Autodesk Inventor part; units mm, degrees
(part 6 of 8)
  spline S746 degree 2 poles (-18.7329, -20.1182) (-18.7329, -19.7747) (-18.2437, -19.289) (-17.9037, -19.289) knots 0 0 0 1 2 2 2
  line L2512 (-18.7329, -20.1182) -> (-18.7329, -19.7747) construction
  line L2513 (-18.7329, -19.7747) -> (-18.2437, -19.289) construction
  line L2514 (-18.2437, -19.289) -> (-17.9037, -19.289) construction
  line L2515 (-17.9037, -19.289) -> (-16.8664, -19.289)
  spline S747 degree 2 poles (-16.8664, -19.289) (-16.6582, -19.289) (-16.6582, -19.4972) knots 0 0 0 1 1 1
  line L2516 (-16.8664, -19.289) -> (-16.6582, -19.289) construction
  line L2517 (-16.6582, -19.289) -> (-16.6582, -19.4972) construction
  line L2518 (-16.6582, -19.4972) -> (-16.6582, -21.3602)
  spline S748 degree 2 poles (-16.6582, -21.3602) (-16.6582, -21.6725) (-16.3668, -21.7974) knots 0 0 0 1 1 1
  line L2519 (-16.6582, -21.3602) -> (-16.6582, -21.6725) construction
  line L2520 (-16.6582, -21.6725) -> (-16.3668, -21.7974) construction
  spline S749 degree 2 poles (-16.3668, -21.7974) (-16.2384, -21.8494) (-16.2384, -21.9812) knots 0 0 0 1 1 1
  line L2521 (-16.3668, -21.7974) -> (-16.2384, -21.8494) construction
  line L2522 (-16.2384, -21.8494) -> (-16.2384, -21.9812) construction
  spline S750 degree 2 poles (-16.2384, -21.9812) (-16.2384, -22.068) (-16.3564, -22.1998) (-16.4431, -22.1998) knots 0 0 0 1 2 2 2
  line L2523 (-16.2384, -21.9812) -> (-16.2384, -22.068) construction
  line L2524 (-16.2384, -22.068) -> (-16.3564, -22.1998) construction
  line L2525 (-16.3564, -22.1998) -> (-16.4431, -22.1998) construction
  spline S751 degree 2 poles (-16.4431, -22.1998) (-16.4882, -22.1998) (-16.5333, -22.179) knots 0 0 0 1 1 1
  line L2526 (-16.4431, -22.1998) -> (-16.4882, -22.1998) construction
  line L2527 (-16.4882, -22.1998) -> (-16.5333, -22.179) construction
  spline S752 degree 2 poles (-16.5333, -22.179) (-16.7415, -22.0888) (-16.8699, -21.9222) knots 0 0 0 1 1 1
  line L2528 (-16.5333, -22.179) -> (-16.7415, -22.0888) construction
  line L2529 (-16.7415, -22.0888) -> (-16.8699, -21.9222) construction
  spline S753 degree 2 poles (-16.8699, -21.9222) (-17.1197, -22.1963) (-17.4874, -22.1963) knots 0 0 0 1 1 1
  line L2530 (-16.8699, -21.9222) -> (-17.1197, -22.1963) construction
  line L2531 (-17.1197, -22.1963) -> (-17.4874, -22.1963) construction
  spline S754 degree 2 poles (-13.9591, -22.1963) (-14.1673, -22.1963) (-14.1673, -21.9882) knots 0 0 0 1 1 1
  line L2532 (-13.9591, -22.1963) -> (-14.1673, -22.1963) construction
  line L2533 (-14.1673, -22.1963) -> (-14.1673, -21.9882) construction
  line L2534 (-14.1673, -21.9882) -> (-14.1673, -20.1217)
  spline S755 degree 2 poles (-14.1673, -20.1217) (-14.1673, -19.9517) (-14.4101, -19.7053) (-14.5801, -19.7053) knots 0 0 0 1 2 2 2
  line L2535 (-14.1673, -20.1217) -> (-14.1673, -19.9517) construction
  line L2536 (-14.1673, -19.9517) -> (-14.4101, -19.7053) construction
  line L2537 (-14.4101, -19.7053) -> (-14.5801, -19.7053) construction
  spline S756 degree 2 poles (-15.4093, -21.9882) (-15.4093, -22.1963) (-15.6174, -22.1963) knots 0 0 0 1 1 1
  line L2538 (-15.4093, -21.9882) -> (-15.4093, -22.1963) construction
  line L2539 (-15.4093, -22.1963) -> (-15.6174, -22.1963) construction
  spline S757 degree 2 poles (-15.6174, -22.1963) (-15.8256, -22.1963) (-15.8256, -21.9882) knots 0 0 0 1 1 1
  line L2540 (-15.6174, -22.1963) -> (-15.8256, -22.1963) construction
  line L2541 (-15.8256, -22.1963) -> (-15.8256, -21.9882) construction
  line L2542 (-15.8256, -21.9882) -> (-15.8256, -19.4972)
  spline S758 degree 2 poles (-15.8256, -19.4972) (-15.8256, -19.289) (-15.6174, -19.289) knots 0 0 0 1 1 1
  line L2543 (-15.8256, -19.4972) -> (-15.8256, -19.289) construction
  line L2544 (-15.8256, -19.289) -> (-15.6174, -19.289) construction
  line L2545 (-15.6174, -19.289) -> (-14.5801, -19.289)
  spline S759 degree 2 poles (-14.5801, -19.289) (-14.2366, -19.289) (-13.7509, -19.7747) (-13.7509, -20.1182) knots 0 0 0 1 2 2 2
  line L2546 (-14.5801, -19.289) -> (-14.2366, -19.289) construction
  line L2547 (-14.2366, -19.289) -> (-13.7509, -19.7747) construction
  line L2548 (-13.7509, -19.7747) -> (-13.7509, -20.1182) construction
  line L2549 (-13.7509, -20.1182) -> (-13.7509, -21.9882)
  spline S760 degree 2 poles (-13.7509, -21.9882) (-13.7509, -22.1963) (-13.9591, -22.1963) knots 0 0 0 1 1 1
  line L2550 (-13.7509, -21.9882) -> (-13.7509, -22.1963) construction
  line L2551 (-13.7509, -22.1963) -> (-13.9591, -22.1963) construction
  spline S761 degree 2 poles (-9.1784, -22.1963) (-9.5184, -22.1963) (-10.011, -21.7106) (-10.011, -21.3672) knots 0 0 0 1 2 2 2
  line L2552 (-9.1784, -22.1963) -> (-9.5184, -22.1963) construction
  line L2553 (-9.5184, -22.1963) -> (-10.011, -21.7106) construction
  line L2554 (-10.011, -21.7106) -> (-10.011, -21.3672) construction
  line L2555 (-10.011, -21.3672) -> (-10.011, -20.1182)
  spline S762 degree 2 poles (-10.011, -20.1182) (-10.011, -19.7747) (-9.5184, -19.289) (-9.1784, -19.289) knots 0 0 0 1 2 2 2
  line L2556 (-10.011, -20.1182) -> (-10.011, -19.7747) construction
  line L2557 (-10.011, -19.7747) -> (-9.5184, -19.289) construction
  line L2558 (-9.5184, -19.289) -> (-9.1784, -19.289) construction
  line L2559 (-9.1784, -19.289) -> (-8.5573, -19.289)
  spline S763 degree 2 poles (-8.5573, -19.289) (-8.3492, -19.289) (-8.3492, -19.4972) knots 0 0 0 1 1 1
  line L2560 (-8.5573, -19.289) -> (-8.3492, -19.289) construction
  line L2561 (-8.3492, -19.289) -> (-8.3492, -19.4972) construction
  spline S764 degree 2 poles (-8.3492, -19.4972) (-8.3492, -19.7053) (-8.5573, -19.7053) knots 0 0 0 1 1 1
  line L2562 (-8.3492, -19.4972) -> (-8.3492, -19.7053) construction
  line L2563 (-8.3492, -19.7053) -> (-8.5573, -19.7053) construction
  line L2564 (-8.5573, -19.7053) -> (-9.1784, -19.7053)
  spline S765 degree 2 poles (-9.1784, -19.7053) (-9.3484, -19.7053) (-9.5947, -19.9517) (-9.5947, -20.1217) knots 0 0 0 1 2 2 2
  line L2565 (-9.1784, -19.7053) -> (-9.3484, -19.7053) construction
  line L2566 (-9.3484, -19.7053) -> (-9.5947, -19.9517) construction
  line L2567 (-9.5947, -19.9517) -> (-9.5947, -20.1217) construction
  line L2568 (-9.5947, -20.1217) -> (-9.5947, -21.3637)
  spline S766 degree 2 poles (-9.5947, -21.3637) (-9.5947, -21.5337) (-9.3484, -21.78) (-9.1784, -21.78) knots 0 0 0 1 2 2 2
  line L2569 (-9.5947, -21.3637) -> (-9.5947, -21.5337) construction
  line L2570 (-9.5947, -21.5337) -> (-9.3484, -21.78) construction
  line L2571 (-9.3484, -21.78) -> (-9.1784, -21.78) construction
  line L2572 (-9.1784, -21.78) -> (-8.5573, -21.78)
  spline S767 degree 2 poles (-8.5573, -21.78) (-8.3492, -21.78) (-8.3492, -21.9882) knots 0 0 0 1 1 1
  line L2573 (-8.5573, -21.78) -> (-8.3492, -21.78) construction
  line L2574 (-8.3492, -21.78) -> (-8.3492, -21.9882) construction
  spline S768 degree 2 poles (-8.3492, -21.9882) (-8.3492, -22.1963) (-8.5573, -22.1963) knots 0 0 0 1 1 1
  line L2575 (-8.3492, -21.9882) -> (-8.3492, -22.1963) construction
  line L2576 (-8.3492, -22.1963) -> (-8.5573, -22.1963) construction
  line L2577 (-8.5573, -22.1963) -> (-9.1784, -22.1963)
  spline S769 degree 2 poles (-17.474, -28.914) (-17.2173, -28.914) (-16.853, -28.5497) (-16.853, -28.293) knots 0 0 0 1 2 2 2
  line L2578 (-17.474, -28.914) -> (-17.2173, -28.914) construction
  line L2579 (-17.2173, -28.914) -> (-16.853, -28.5497) construction
  line L2580 (-16.853, -28.5497) -> (-16.853, -28.293) construction
  line L2581 (-16.853, -28.293) -> (-16.853, -26.2149)
  spline S770 degree 2 poles (-16.853, -26.2149) (-16.853, -25.9581) (-17.2173, -25.5939) (-17.474, -25.5939) knots 0 0 0 1 2 2 2
  line L2582 (-16.853, -26.2149) -> (-16.853, -25.9581) construction
  line L2583 (-16.853, -25.9581) -> (-17.2173, -25.5939) construction
  line L2584 (-17.2173, -25.5939) -> (-17.474, -25.5939) construction
  line L2585 (-17.474, -29.3303) -> (-18.7195, -29.3303)
  spline S771 degree 2 poles (-18.7195, -29.3303) (-18.8028, -29.3303) (-18.9277, -29.2054) (-18.9277, -29.1222) knots 0 0 0 1 2 2 2
  line L2586 (-18.7195, -29.3303) -> (-18.8028, -29.3303) construction
  line L2587 (-18.8028, -29.3303) -> (-18.9277, -29.2054) construction
  line L2588 (-18.9277, -29.2054) -> (-18.9277, -29.1222) construction
  line L2589 (-18.9277, -29.1222) -> (-18.9277, -25.3857)
  spline S772 degree 2 poles (-18.9277, -25.3857) (-18.9277, -25.3024) (-18.8028, -25.1775) (-18.7195, -25.1775) knots 0 0 0 1 2 2 2
  line L2590 (-18.9277, -25.3857) -> (-18.9277, -25.3024) construction
  line L2591 (-18.9277, -25.3024) -> (-18.8028, -25.1775) construction
  line L2592 (-18.8028, -25.1775) -> (-18.7195, -25.1775) construction
  line L2593 (-18.7195, -25.1775) -> (-17.474, -25.1775)
  spline S773 degree 2 poles (-17.474, -25.1775) (-17.0438, -25.1775) (-16.4367, -25.7881) (-16.4367, -26.2149) knots 0 0 0 1 2 2 2
  line L2594 (-17.474, -25.1775) -> (-17.0438, -25.1775) construction
  line L2595 (-17.0438, -25.1775) -> (-16.4367, -25.7881) construction
  line L2596 (-16.4367, -25.7881) -> (-16.4367, -26.2149) construction
  line L2597 (-16.4367, -26.2149) -> (-16.4367, -28.293)
  spline S774 degree 2 poles (-16.4367, -28.293) (-16.4367, -28.7232) (-17.0438, -29.3303) (-17.474, -29.3303) knots 0 0 0 1 2 2 2
  line L2598 (-16.4367, -28.293) -> (-16.4367, -28.7232) construction
  line L2599 (-16.4367, -28.7232) -> (-17.0438, -29.3303) construction
  line L2600 (-17.0438, -29.3303) -> (-17.474, -29.3303) construction
  spline S775 degree 2 poles (-19.6338, -32.3113) (-19.4256, -32.3113) (-19.4256, -32.5194) knots 0 0 0 1 1 1
  line L2601 (-19.6338, -32.3113) -> (-19.4256, -32.3113) construction
  line L2602 (-19.4256, -32.3113) -> (-19.4256, -32.5194) construction
  spline S776 degree 2 poles (-19.4256, -32.5194) (-19.4256, -32.7276) (-19.6338, -32.7276) knots 0 0 0 1 1 1
  line L2603 (-19.4256, -32.5194) -> (-19.4256, -32.7276) construction
  line L2604 (-19.4256, -32.7276) -> (-19.6338, -32.7276) construction
  spline S777 degree 2 poles (-21.0874, -34.601) (-21.0874, -34.8092) (-21.2956, -34.8092) knots 0 0 0 1 1 1
  line L2605 (-21.0874, -34.601) -> (-21.0874, -34.8092) construction
  line L2606 (-21.0874, -34.8092) -> (-21.2956, -34.8092) construction
  spline S778 degree 2 poles (-21.2956, -34.8092) (-21.5037, -34.8092) (-21.5037, -34.601) knots 0 0 0 1 1 1
  line L2607 (-21.2956, -34.8092) -> (-21.5037, -34.8092) construction
  line L2608 (-21.5037, -34.8092) -> (-21.5037, -34.601) construction
  line L2609 (-21.5037, -34.601) -> (-21.5037, -30.8646)
  spline S779 degree 2 poles (-21.5037, -30.8646) (-21.5037, -30.6564) (-21.2956, -30.6564) knots 0 0 0 1 1 1
  line L2610 (-21.5037, -30.8646) -> (-21.5037, -30.6564) construction
  line L2611 (-21.5037, -30.6564) -> (-21.2956, -30.6564) construction
  line L2612 (-21.2956, -30.6564) -> (-19.6338, -30.6564)
  spline S780 degree 2 poles (-19.6338, -30.6564) (-19.4256, -30.6564) (-19.4256, -30.8646) knots 0 0 0 1 1 1
  line L2613 (-19.6338, -30.6564) -> (-19.4256, -30.6564) construction
  line L2614 (-19.4256, -30.6564) -> (-19.4256, -30.8646) construction
  spline S781 degree 2 poles (-19.4256, -30.8646) (-19.4256, -31.0727) (-19.6338, -31.0727) knots 0 0 0 1 1 1
  line L2615 (-19.4256, -30.8646) -> (-19.4256, -31.0727) construction
  line L2616 (-19.4256, -31.0727) -> (-19.6338, -31.0727) construction
  line L2617 (9.3223, -22.1486) -> (8.2849, -22.1486)
  spline S782 degree 2 poles (8.2849, -22.1486) (7.9449, -22.1486) (7.4558, -21.6629) (7.4558, -21.3195) knots 0 0 0 1 2 2 2
  line L2618 (8.2849, -22.1486) -> (7.9449, -22.1486) construction
  line L2619 (7.9449, -22.1486) -> (7.4558, -21.6629) construction
  line L2620 (7.4558, -21.6629) -> (7.4558, -21.3195) construction
  line L2621 (7.4558, -21.3195) -> (7.4558, -19.4495)
  spline S783 degree 2 poles (7.4558, -19.4495) (7.4558, -19.2413) (7.6639, -19.2413) knots 0 0 0 1 1 1
  line L2622 (7.4558, -19.4495) -> (7.4558, -19.2413) construction
  line L2623 (7.4558, -19.2413) -> (7.6639, -19.2413) construction
  spline S784 degree 2 poles (7.6639, -19.2413) (7.8721, -19.2413) (7.8721, -19.4495) knots 0 0 0 1 1 1
  line L2624 (7.6639, -19.2413) -> (7.8721, -19.2413) construction
  line L2625 (7.8721, -19.2413) -> (7.8721, -19.4495) construction
  line L2626 (7.8721, -19.4495) -> (7.8721, -21.316)
  spline S785 degree 2 poles (7.8721, -21.316) (7.8721, -21.486) (8.1149, -21.7323) (8.2849, -21.7323) knots 0 0 0 1 2 2 2
  line L2627 (7.8721, -21.316) -> (7.8721, -21.486) construction
  line L2628 (7.8721, -21.486) -> (8.1149, -21.7323) construction
  line L2629 (8.1149, -21.7323) -> (8.2849, -21.7323) construction
  spline S786 degree 2 poles (9.1141, -19.4495) (9.1141, -19.2413) (9.3223, -19.2413) knots 0 0 0 1 1 1
  line L2630 (9.1141, -19.4495) -> (9.1141, -19.2413) construction
  line L2631 (9.1141, -19.2413) -> (9.3223, -19.2413) construction
  spline S787 degree 2 poles (9.3223, -19.2413) (9.5304, -19.2413) (9.5304, -19.4495) knots 0 0 0 1 1 1
  line L2632 (9.3223, -19.2413) -> (9.5304, -19.2413) construction
  line L2633 (9.5304, -19.2413) -> (9.5304, -19.4495) construction
  line L2634 (9.5304, -19.4495) -> (9.5304, -21.9405)
  spline S788 degree 2 poles (9.5304, -21.9405) (9.5304, -22.1486) (9.3223, -22.1486) knots 0 0 0 1 1 1
  line L2635 (9.5304, -21.9405) -> (9.5304, -22.1486) construction
  line L2636 (9.5304, -22.1486) -> (9.3223, -22.1486) construction
  spline S789 degree 2 poles (15.345, -22.1486) (15.1369, -22.1486) (15.1369, -21.9405) knots 0 0 0 1 1 1
  line L2637 (15.345, -22.1486) -> (15.1369, -22.1486) construction
  line L2638 (15.1369, -22.1486) -> (15.1369, -21.9405) construction
  spline S790 degree 2 poles (14.4777, -21.0211) (14.3979, -21.1356) (14.3077, -21.1356) knots 0 0 0 1 1 1
  line L2639 (14.4777, -21.0211) -> (14.3979, -21.1356) construction
  line L2640 (14.3979, -21.1356) -> (14.3077, -21.1356) construction
  spline S791 degree 2 poles (14.3077, -21.1356) (14.2175, -21.1356) (14.1377, -21.0211) knots 0 0 0 1 1 1
  line L2641 (14.3077, -21.1356) -> (14.2175, -21.1356) construction
  line L2642 (14.2175, -21.1356) -> (14.1377, -21.0211) construction
  spline S792 degree 2 poles (13.4785, -21.9405) (13.4785, -22.1486) (13.2704, -22.1486) knots 0 0 0 1 1 1
  line L2643 (13.4785, -21.9405) -> (13.4785, -22.1486) construction
  line L2644 (13.4785, -22.1486) -> (13.2704, -22.1486) construction
  spline S793 degree 2 poles (13.2704, -22.1486) (13.0622, -22.1486) (13.0622, -21.9405) knots 0 0 0 1 1 1
  line L2645 (13.2704, -22.1486) -> (13.0622, -22.1486) construction
  line L2646 (13.0622, -22.1486) -> (13.0622, -21.9405) construction
  line L2647 (13.0622, -21.9405) -> (13.0622, -19.446)
  spline S794 degree 2 poles (13.0622, -19.446) (13.0622, -19.2066) (13.2461, -19.2066) knots 0 0 0 1 1 1
  line L2648 (13.0622, -19.446) -> (13.0622, -19.2066) construction
  line L2649 (13.0622, -19.2066) -> (13.2461, -19.2066) construction
  spline S795 degree 2 poles (13.2461, -19.2066) (13.3536, -19.2066) (13.4404, -19.3281) knots 0 0 0 1 1 1
  line L2650 (13.2461, -19.2066) -> (13.3536, -19.2066) construction
  line L2651 (13.3536, -19.2066) -> (13.4404, -19.3281) construction
  spline S796 degree 2 poles (15.175, -19.3281) (15.2618, -19.2066) (15.3693, -19.2066) knots 0 0 0 1 1 1
  line L2652 (15.175, -19.3281) -> (15.2618, -19.2066) construction
  line L2653 (15.2618, -19.2066) -> (15.3693, -19.2066) construction
  spline S797 degree 2 poles (15.3693, -19.2066) (15.5532, -19.2066) (15.5532, -19.446) knots 0 0 0 1 1 1
  line L2654 (15.3693, -19.2066) -> (15.5532, -19.2066) construction
  line L2655 (15.5532, -19.2066) -> (15.5532, -19.446) construction
  line L2656 (15.5532, -19.446) -> (15.5532, -21.9405)
  spline S798 degree 2 poles (15.5532, -21.9405) (15.5532, -22.1486) (15.345, -22.1486) knots 0 0 0 1 1 1
  line L2657 (15.5532, -21.9405) -> (15.5532, -22.1486) construction
  line L2658 (15.5532, -22.1486) -> (15.345, -22.1486) construction
  spline S799 degree 2 poles (6.716, -26.7765) (6.886, -26.7765) (7.1288, -26.5301) (7.1288, -26.3601) knots 0 0 0 1 2 2 2
  line L2659 (6.716, -26.7765) -> (6.886, -26.7765) construction
  line L2660 (6.886, -26.7765) -> (7.1288, -26.5301) construction
  line L2661 (7.1288, -26.5301) -> (7.1288, -26.3601) construction
  line L2662 (7.1288, -26.3601) -> (7.1288, -25.1181)
  spline S800 degree 2 poles (7.1288, -25.1181) (7.1288, -24.9481) (6.886, -24.7018) (6.716, -24.7018) knots 0 0 0 1 2 2 2
  line L2663 (7.1288, -25.1181) -> (7.1288, -24.9481) construction
  line L2664 (7.1288, -24.9481) -> (6.886, -24.7018) construction
  line L2665 (6.886, -24.7018) -> (6.716, -24.7018) construction
  line L2666 (6.716, -24.7018) -> (6.2997, -24.7018)
  spline S801 degree 2 poles (6.2997, -24.7018) (6.1297, -24.7018) (5.8868, -24.9481) (5.8868, -25.1181) knots 0 0 0 1 2 2 2
  line L2667 (6.2997, -24.7018) -> (6.1297, -24.7018) construction
  line L2668 (6.1297, -24.7018) -> (5.8868, -24.9481) construction
  line L2669 (5.8868, -24.9481) -> (5.8868, -25.1181) construction
  line L2670 (5.8868, -25.1181) -> (5.8868, -26.3601)
  spline S802 degree 2 poles (5.8868, -26.3601) (5.8868, -26.5301) (6.1297, -26.7765) (6.2997, -26.7765) knots 0 0 0 1 2 2 2
  line L2671 (5.8868, -26.3601) -> (5.8868, -26.5301) construction
  line L2672 (5.8868, -26.5301) -> (6.1297, -26.7765) construction
  line L2673 (6.1297, -26.7765) -> (6.2997, -26.7765) construction
  line L2674 (6.2997, -26.7765) -> (6.716, -26.7765)
  spline S803 degree 2 poles (5.5329, -23.3973) (5.4566, -23.321) (5.4566, -23.2273) knots 0 0 0 1 1 1
  line L2675 (5.5329, -23.3973) -> (5.4566, -23.321) construction
  line L2676 (5.4566, -23.321) -> (5.4566, -23.2273) construction
  spline S804 degree 2 poles (5.4566, -23.2273) (5.4566, -23.04) (5.6752, -23.04) knots 0 0 0 1 1 1
  line L2677 (5.4566, -23.2273) -> (5.4566, -23.04) construction
  line L2678 (5.4566, -23.04) -> (5.6752, -23.04) construction
  line L2679 (5.6752, -23.04) -> (7.337, -23.04)
  spline S805 degree 2 poles (7.337, -23.04) (7.5452, -23.04) (7.5452, -23.2482) knots 0 0 0 1 1 1
  line L2680 (7.337, -23.04) -> (7.5452, -23.04) construction
  line L2681 (7.5452, -23.04) -> (7.5452, -23.2482) construction
  spline S806 degree 2 poles (7.5452, -23.2482) (7.5452, -23.4563) (7.337, -23.4563) knots 0 0 0 1 1 1
  line L2682 (7.5452, -23.2482) -> (7.5452, -23.4563) construction
  line L2683 (7.5452, -23.4563) -> (7.337, -23.4563) construction
  spline S807 degree 2 poles (7.2954, -24.5075) (7.3301, -24.5353) (7.3474, -24.5734) knots 0 0 0 1 1 1
  line L2684 (7.2954, -24.5075) -> (7.3301, -24.5353) construction
  line L2685 (7.3301, -24.5353) -> (7.3474, -24.5734) construction
  spline S808 degree 2 poles (7.3474, -24.5734) (7.5452, -24.8059) (7.5452, -25.1181) knots 0 0 0 1 1 1
  line L2686 (7.3474, -24.5734) -> (7.5452, -24.8059) construction
  line L2687 (7.5452, -24.8059) -> (7.5452, -25.1181) construction
  line L2688 (7.5452, -25.1181) -> (7.5452, -26.3636)
  spline S809 degree 2 poles (7.5452, -26.3636) (7.5452, -26.7071) (7.0594, -27.1928) (6.716, -27.1928) knots 0 0 0 1 2 2 2
  line L2689 (7.5452, -26.3636) -> (7.5452, -26.7071) construction
  line L2690 (7.5452, -26.7071) -> (7.0594, -27.1928) construction
  line L2691 (7.0594, -27.1928) -> (6.716, -27.1928) construction
  line L2692 (6.716, -27.1928) -> (6.2997, -27.1928)
  spline S810 degree 2 poles (6.2997, -27.1928) (5.9597, -27.1928) (5.4705, -26.7071) (5.4705, -26.3636) knots 0 0 0 1 2 2 2
  line L2693 (6.2997, -27.1928) -> (5.9597, -27.1928) construction
  line L2694 (5.9597, -27.1928) -> (5.4705, -26.7071) construction
  line L2695 (5.4705, -26.7071) -> (5.4705, -26.3636) construction
  line L2696 (5.4705, -26.3636) -> (5.4705, -25.1147)
  spline S811 degree 2 poles (5.4705, -25.1147) (5.4705, -24.7712) (5.9597, -24.2855) (6.2997, -24.2855) knots 0 0 0 1 2 2 2
  line L2697 (5.4705, -25.1147) -> (5.4705, -24.7712) construction
  line L2698 (5.4705, -24.7712) -> (5.9597, -24.2855) construction
  line L2699 (5.9597, -24.2855) -> (6.2997, -24.2855) construction
  spline S812 degree 2 poles (9.6233, -26.7765) (9.7933, -26.7765) (10.0361, -26.5301) (10.0361, -26.3601) knots 0 0 0 1 2 2 2
  line L2700 (9.6233, -26.7765) -> (9.7933, -26.7765) construction
  line L2701 (9.7933, -26.7765) -> (10.0361, -26.5301) construction
  line L2702 (10.0361, -26.5301) -> (10.0361, -26.3601) construction
  spline S813 degree 2 poles (9.207, -24.7018) (9.037, -24.7018) (8.7941, -24.9481) (8.7941, -25.1181) knots 0 0 0 1 2 2 2
  line L2703 (9.207, -24.7018) -> (9.037, -24.7018) construction
  line L2704 (9.037, -24.7018) -> (8.7941, -24.9481) construction
  line L2705 (8.7941, -24.9481) -> (8.7941, -25.1181) construction
  line L2706 (8.7941, -25.1181) -> (8.7941, -26.3601)
  spline S814 degree 2 poles (8.7941, -26.3601) (8.7941, -26.5301) (9.037, -26.7765) (9.207, -26.7765) knots 0 0 0 1 2 2 2
  line L2707 (8.7941, -26.3601) -> (8.7941, -26.5301) construction
  line L2708 (8.7941, -26.5301) -> (9.037, -26.7765) construction
  line L2709 (9.037, -26.7765) -> (9.207, -26.7765) construction
  line L2710 (9.207, -26.7765) -> (9.6233, -26.7765)
  line L2711 (9.6233, -27.1928) -> (9.207, -27.1928)
  spline S815 degree 2 poles (9.207, -27.1928) (8.867, -27.1928) (8.3778, -26.7071) (8.3778, -26.3636) knots 0 0 0 1 2 2 2
  line L2712 (9.207, -27.1928) -> (8.867, -27.1928) construction
  line L2713 (8.867, -27.1928) -> (8.3778, -26.7071) construction
  line L2714 (8.3778, -26.7071) -> (8.3778, -26.3636) construction
  line L2715 (8.3778, -26.3636) -> (8.3778, -25.1147)
  spline S816 degree 2 poles (8.3778, -25.1147) (8.3778, -24.7712) (8.867, -24.2855) (9.207, -24.2855) knots 0 0 0 1 2 2 2
  line L2716 (8.3778, -25.1147) -> (8.3778, -24.7712) construction
  line L2717 (8.3778, -24.7712) -> (8.867, -24.2855) construction
  line L2718 (8.867, -24.2855) -> (9.207, -24.2855) construction
  line L2719 (9.207, -24.2855) -> (10.2443, -24.2855)
  spline S817 degree 2 poles (10.2443, -24.2855) (10.4524, -24.2855) (10.4524, -24.4936) knots 0 0 0 1 1 1
  line L2720 (10.2443, -24.2855) -> (10.4524, -24.2855) construction
  line L2721 (10.4524, -24.2855) -> (10.4524, -24.4936) construction
  line L2722 (10.4524, -24.4936) -> (10.4524, -26.3567)
  spline S818 degree 2 poles (10.4524, -26.3567) (10.4524, -26.6689) (10.7439, -26.7938) knots 0 0 0 1 1 1
  line L2723 (10.4524, -26.3567) -> (10.4524, -26.6689) construction
  line L2724 (10.4524, -26.6689) -> (10.7439, -26.7938) construction
  spline S819 degree 2 poles (10.7439, -26.7938) (10.8722, -26.8459) (10.8722, -26.9777) knots 0 0 0 1 1 1
  line L2725 (10.7439, -26.7938) -> (10.8722, -26.8459) construction
  line L2726 (10.8722, -26.8459) -> (10.8722, -26.9777) construction
  spline S820 degree 2 poles (10.8722, -26.9777) (10.8722, -27.0644) (10.7543, -27.1963) (10.6675, -27.1963) knots 0 0 0 1 2 2 2
  line L2727 (10.8722, -26.9777) -> (10.8722, -27.0644) construction
  line L2728 (10.8722, -27.0644) -> (10.7543, -27.1963) construction
  line L2729 (10.7543, -27.1963) -> (10.6675, -27.1963) construction
  spline S821 degree 2 poles (10.6675, -27.1963) (10.6224, -27.1963) (10.5773, -27.1754) knots 0 0 0 1 1 1
  line L2730 (10.6675, -27.1963) -> (10.6224, -27.1963) construction
  line L2731 (10.6224, -27.1963) -> (10.5773, -27.1754) construction
  spline S822 degree 2 poles (10.5773, -27.1754) (10.3692, -27.0852) (10.2408, -26.9187) knots 0 0 0 1 1 1
  line L2732 (10.5773, -27.1754) -> (10.3692, -27.0852) construction
  line L2733 (10.3692, -27.0852) -> (10.2408, -26.9187) construction
  spline S823 degree 2 poles (10.2408, -26.9187) (9.991, -27.1928) (9.6233, -27.1928) knots 0 0 0 1 1 1
  line L2734 (10.2408, -26.9187) -> (9.991, -27.1928) construction
  line L2735 (9.991, -27.1928) -> (9.6233, -27.1928) construction
  spline S824 degree 2 poles (12.5306, -26.7765) (12.7006, -26.7765) (12.9434, -26.5301) (12.9434, -26.3601) knots 0 0 0 1 2 2 2
  line L2736 (12.5306, -26.7765) -> (12.7006, -26.7765) construction
  line L2737 (12.7006, -26.7765) -> (12.9434, -26.5301) construction
  line L2738 (12.9434, -26.5301) -> (12.9434, -26.3601) construction
  line L2739 (12.9434, -26.3601) -> (12.9434, -25.1181)
  spline S825 degree 2 poles (12.9434, -25.1181) (12.9434, -24.9481) (12.7006, -24.7018) (12.5306, -24.7018) knots 0 0 0 1 2 2 2
  line L2740 (12.9434, -25.1181) -> (12.9434, -24.9481) construction
  line L2741 (12.9434, -24.9481) -> (12.7006, -24.7018) construction
  line L2742 (12.7006, -24.7018) -> (12.5306, -24.7018) construction
  spline S826 degree 2 poles (11.7014, -28.2301) (11.7014, -28.4383) (11.4932, -28.4383) knots 0 0 0 1 1 1
  line L2743 (11.7014, -28.2301) -> (11.7014, -28.4383) construction
  line L2744 (11.7014, -28.4383) -> (11.4932, -28.4383) construction
  spline S827 degree 2 poles (11.4932, -28.4383) (11.2851, -28.4383) (11.2851, -28.2301) knots 0 0 0 1 1 1
  line L2745 (11.4932, -28.4383) -> (11.2851, -28.4383) construction
  line L2746 (11.2851, -28.4383) -> (11.2851, -28.2301) construction
  line L2747 (11.2851, -28.2301) -> (11.2851, -24.4936)
  spline S828 degree 2 poles (11.2851, -24.4936) (11.2851, -24.2855) (11.4932, -24.2855) knots 0 0 0 1 1 1
  line L2748 (11.2851, -24.4936) -> (11.2851, -24.2855) construction
  line L2749 (11.2851, -24.2855) -> (11.4932, -24.2855) construction
  line L2750 (11.4932, -24.2855) -> (12.5306, -24.2855)
  spline S829 degree 2 poles (12.5306, -24.2855) (12.874, -24.2855) (13.3597, -24.7712) (13.3597, -25.1147) knots 0 0 0 1 2 2 2
  line L2751 (12.5306, -24.2855) -> (12.874, -24.2855) construction
  line L2752 (12.874, -24.2855) -> (13.3597, -24.7712) construction
  line L2753 (13.3597, -24.7712) -> (13.3597, -25.1147) construction
  line L2754 (13.3597, -25.1147) -> (13.3597, -26.3636)
  spline S830 degree 2 poles (13.3597, -26.3636) (13.3597, -26.7071) (12.874, -27.1928) (12.5306, -27.1928) knots 0 0 0 1 2 2 2
  line L2755 (13.3597, -26.3636) -> (13.3597, -26.7071) construction
  line L2756 (13.3597, -26.7071) -> (12.874, -27.1928) construction
  line L2757 (12.874, -27.1928) -> (12.5306, -27.1928) construction
  spline S831 degree 2 poles (6.6613, -33.0115) (6.8313, -33.0115) (7.0741, -32.7652) (7.0741, -32.5952) knots 0 0 0 1 2 2 2
  line L2758 (6.6613, -33.0115) -> (6.8313, -33.0115) construction
  line L2759 (6.8313, -33.0115) -> (7.0741, -32.7652) construction
  line L2760 (7.0741, -32.7652) -> (7.0741, -32.5952) construction
  spline S832 degree 2 poles (6.245, -30.9369) (6.075, -30.9369) (5.8321, -31.1832) (5.8321, -31.3532) knots 0 0 0 1 2 2 2
  line L2761 (6.245, -30.9369) -> (6.075, -30.9369) construction
  line L2762 (6.075, -30.9369) -> (5.8321, -31.1832) construction
  line L2763 (5.8321, -31.1832) -> (5.8321, -31.3532) construction
  line L2764 (5.8321, -31.3532) -> (5.8321, -32.5952)
  spline S833 degree 2 poles (5.8321, -32.5952) (5.8321, -32.7652) (6.075, -33.0115) (6.245, -33.0115) knots 0 0 0 1 2 2 2
  line L2765 (5.8321, -32.5952) -> (5.8321, -32.7652) construction
  line L2766 (5.8321, -32.7652) -> (6.075, -33.0115) construction
  line L2767 (6.075, -33.0115) -> (6.245, -33.0115) construction
  line L2768 (6.245, -33.0115) -> (6.6613, -33.0115)
  line L2769 (6.6613, -33.4278) -> (6.245, -33.4278)
  spline S834 degree 2 poles (6.245, -33.4278) (5.905, -33.4278) (5.4158, -32.9421) (5.4158, -32.5987) knots 0 0 0 1 2 2 2
  line L2770 (6.245, -33.4278) -> (5.905, -33.4278) construction
  line L2771 (5.905, -33.4278) -> (5.4158, -32.9421) construction
  line L2772 (5.4158, -32.9421) -> (5.4158, -32.5987) construction
  line L2773 (5.4158, -32.5987) -> (5.4158, -31.3497)
  spline S835 degree 2 poles (5.4158, -31.3497) (5.4158, -31.0062) (5.905, -30.5205) (6.245, -30.5205) knots 0 0 0 1 2 2 2
  line L2774 (5.4158, -31.3497) -> (5.4158, -31.0062) construction
  line L2775 (5.4158, -31.0062) -> (5.905, -30.5205) construction
  line L2776 (5.905, -30.5205) -> (6.245, -30.5205) construction
  line L2777 (6.245, -30.5205) -> (7.2823, -30.5205)
  spline S836 degree 2 poles (7.2823, -30.5205) (7.4904, -30.5205) (7.4904, -30.7287) knots 0 0 0 1 1 1
  line L2778 (7.2823, -30.5205) -> (7.4904, -30.5205) construction
  line L2779 (7.4904, -30.5205) -> (7.4904, -30.7287) construction
  line L2780 (7.4904, -30.7287) -> (7.4904, -32.5917)
  spline S837 degree 2 poles (7.4904, -32.5917) (7.4904, -32.904) (7.7819, -33.0289) knots 0 0 0 1 1 1
  line L2781 (7.4904, -32.5917) -> (7.4904, -32.904) construction
  line L2782 (7.4904, -32.904) -> (7.7819, -33.0289) construction
  spline S838 degree 2 poles (7.7819, -33.0289) (7.9102, -33.0809) (7.9102, -33.2127) knots 0 0 0 1 1 1
  line L2783 (7.7819, -33.0289) -> (7.9102, -33.0809) construction
  line L2784 (7.9102, -33.0809) -> (7.9102, -33.2127) construction
  spline S839 degree 2 poles (7.9102, -33.2127) (7.9102, -33.2995) (7.7923, -33.4313) (7.7055, -33.4313) knots 0 0 0 1 2 2 2
  line L2785 (7.9102, -33.2127) -> (7.9102, -33.2995) construction
  line L2786 (7.9102, -33.2995) -> (7.7923, -33.4313) construction
  line L2787 (7.7923, -33.4313) -> (7.7055, -33.4313) construction
  spline S840 degree 2 poles (7.7055, -33.4313) (7.6604, -33.4313) (7.6153, -33.4105) knots 0 0 0 1 1 1
  line L2788 (7.7055, -33.4313) -> (7.6604, -33.4313) construction
  line L2789 (7.6604, -33.4313) -> (7.6153, -33.4105) construction
  spline S841 degree 2 poles (7.6153, -33.4105) (7.4072, -33.3203) (7.2788, -33.1538) knots 0 0 0 1 1 1
  line L2790 (7.6153, -33.4105) -> (7.4072, -33.3203) construction
  line L2791 (7.4072, -33.3203) -> (7.2788, -33.1538) construction
  spline S842 degree 2 poles (7.2788, -33.1538) (7.029, -33.4278) (6.6613, -33.4278) knots 0 0 0 1 1 1
  line L2792 (7.2788, -33.1538) -> (7.029, -33.4278) construction
  line L2793 (7.029, -33.4278) -> (6.6613, -33.4278) construction
  line L2794 (8.6978, -32.557) -> (8.6978, -33.2197)
  spline S843 degree 2 poles (8.6978, -33.2197) (8.6978, -33.4278) (8.4896, -33.4278) knots 0 0 0 1 1 1
  line L2795 (8.6978, -33.2197) -> (8.6978, -33.4278) construction
  line L2796 (8.6978, -33.4278) -> (8.4896, -33.4278) construction
  spline S844 degree 2 poles (8.4896, -33.4278) (8.2815, -33.4278) (8.2815, -33.2197) knots 0 0 0 1 1 1
  line L2797 (8.4896, -33.4278) -> (8.2815, -33.4278) construction
  line L2798 (8.2815, -33.4278) -> (8.2815, -33.2197) construction
  line L2799 (8.2815, -33.2197) -> (8.2815, -30.7287)
  spline S845 degree 2 poles (8.2815, -30.7287) (8.2815, -30.5205) (8.4896, -30.5205) knots 0 0 0 1 1 1
  line L2800 (8.2815, -30.7287) -> (8.2815, -30.5205) construction
  line L2801 (8.2815, -30.5205) -> (8.4896, -30.5205) construction
  spline S846 degree 2 poles (8.4896, -30.5205) (8.6978, -30.5205) (8.6978, -30.7287) knots 0 0 0 1 1 1
  line L2802 (8.4896, -30.5205) -> (8.6978, -30.5205) construction
  line L2803 (8.6978, -30.5205) -> (8.6978, -30.7287) construction
  spline S847 degree 2 poles (10.0161, -30.5691) (10.0716, -30.5067) (10.148, -30.5067) knots 0 0 0 1 1 1
  line L2804 (10.0161, -30.5691) -> (10.0716, -30.5067) construction
  line L2805 (10.0716, -30.5067) -> (10.148, -30.5067) construction
  spline S848 degree 2 poles (10.148, -30.5067) (10.2312, -30.5067) (10.3561, -30.642) (10.3561, -30.7322) knots 0 0 0 1 2 2 2
  line L2806 (10.148, -30.5067) -> (10.2312, -30.5067) construction
  line L2807 (10.2312, -30.5067) -> (10.3561, -30.642) construction
  line L2808 (10.3561, -30.642) -> (10.3561, -30.7322) construction
  spline S849 degree 2 poles (10.3561, -30.7322) (10.3561, -30.8189) (10.2902, -30.8848) knots 0 0 0 1 1 1
  line L2809 (10.3561, -30.7322) -> (10.3561, -30.8189) construction
  line L2810 (10.3561, -30.8189) -> (10.2902, -30.8848) construction
  spline S850 degree 2 poles (10.311, -33.0844) (10.3561, -33.1538) (10.3561, -33.2232) knots 0 0 0 1 1 1
  line L2811 (10.311, -33.0844) -> (10.3561, -33.1538) construction
  line L2812 (10.3561, -33.1538) -> (10.3561, -33.2232) construction
  spline S851 degree 2 poles (10.3561, -33.2232) (10.3561, -33.3099) (10.2208, -33.4348) (10.1445, -33.4348) knots 0 0 0 1 2 2 2
  line L2813 (10.3561, -33.2232) -> (10.3561, -33.3099) construction
  line L2814 (10.3561, -33.3099) -> (10.2208, -33.4348) construction
  line L2815 (10.2208, -33.4348) -> (10.1445, -33.4348) construction
  spline S852 degree 2 poles (10.1445, -33.4348) (10.0473, -33.4348) (9.9953, -33.3515) knots 0 0 0 1 1 1
  line L2816 (10.1445, -33.4348) -> (10.0473, -33.4348) construction
  line L2817 (10.0473, -33.4348) -> (9.9953, -33.3515) construction
  line L2818 (9.9953, -33.3515) -> (9.1627, -32.0679)
  spline S853 degree 2 poles (9.1627, -32.0679) (9.0378, -32.1997) (8.6978, -32.557) knots 0 0 0 1 1 1
  line L2819 (9.1627, -32.0679) -> (9.0378, -32.1997) construction
  line L2820 (9.0378, -32.1997) -> (8.6978, -32.557) construction
  spline S854 degree 2 poles (-18.4295, -40.499) (-18.4295, -40.2909) (-18.2213, -40.2909) knots 0 0 0 1 1 1
  line L2821 (-18.4295, -40.499) -> (-18.4295, -40.2909) construction
  line L2822 (-18.4295, -40.2909) -> (-18.2213, -40.2909) construction
  spline S855 degree 2 poles (-18.2213, -40.2909) (-18.0132, -40.2909) (-18.0132, -40.499) knots 0 0 0 1 1 1
  line L2823 (-18.2213, -40.2909) -> (-18.0132, -40.2909) construction
  line L2824 (-18.0132, -40.2909) -> (-18.0132, -40.499) construction
  line L2825 (-18.0132, -40.499) -> (-18.0132, -42.99)
  spline S856 degree 2 poles (-18.0132, -42.99) (-18.0132, -43.1982) (-18.2213, -43.1982) knots 0 0 0 1 1 1
  line L2826 (-18.0132, -42.99) -> (-18.0132, -43.1982) construction
  line L2827 (-18.0132, -43.1982) -> (-18.2213, -43.1982) construction
  spline S857 degree 2 poles (-18.2213, -43.1982) (-18.4295, -43.1982) (-18.4295, -42.99) knots 0 0 0 1 1 1
  line L2828 (-18.2213, -43.1982) -> (-18.4295, -43.1982) construction
  line L2829 (-18.4295, -43.1982) -> (-18.4295, -42.99) construction
  spline S858 degree 2 poles (-19.6715, -42.99) (-19.6715, -43.1982) (-19.8797, -43.1982) knots 0 0 0 1 1 1
  line L2830 (-19.6715, -42.99) -> (-19.6715, -43.1982) construction
  line L2831 (-19.6715, -43.1982) -> (-19.8797, -43.1982) construction
  spline S859 degree 2 poles (-19.8797, -43.1982) (-20.0878, -43.1982) (-20.0878, -42.99) knots 0 0 0 1 1 1
  line L2832 (-19.8797, -43.1982) -> (-20.0878, -43.1982) construction
  line L2833 (-20.0878, -43.1982) -> (-20.0878, -42.99) construction
  line L2834 (-20.0878, -42.99) -> (-20.0878, -40.499)
  spline S860 degree 2 poles (-20.0878, -40.499) (-20.0878, -40.2909) (-19.8797, -40.2909) knots 0 0 0 1 1 1
  line L2835 (-20.0878, -40.499) -> (-20.0878, -40.2909) construction
  line L2836 (-20.0878, -40.2909) -> (-19.8797, -40.2909) construction
  spline S861 degree 2 poles (-19.8797, -40.2909) (-19.6715, -40.2909) (-19.6715, -40.499) knots 0 0 0 1 1 1
  line L2837 (-19.8797, -40.2909) -> (-19.6715, -40.2909) construction
  line L2838 (-19.6715, -40.2909) -> (-19.6715, -40.499) construction
  spline S862 degree 2 poles (-10.1204, -42.7819) (-9.9504, -42.7819) (-9.7076, -42.5355) (-9.7076, -42.3655) knots 0 0 0 1 2 2 2
  line L2839 (-10.1204, -42.7819) -> (-9.9504, -42.7819) construction
  line L2840 (-9.9504, -42.7819) -> (-9.7076, -42.5355) construction
  line L2841 (-9.7076, -42.5355) -> (-9.7076, -42.3655) construction
  line L2842 (-9.7076, -42.3655) -> (-9.7076, -41.1235)
  spline S863 degree 2 poles (-9.7076, -41.1235) (-9.7076, -40.9535) (-9.9504, -40.7072) (-10.1204, -40.7072) knots 0 0 0 1 2 2 2
  line L2843 (-9.7076, -41.1235) -> (-9.7076, -40.9535) construction
  line L2844 (-9.7076, -40.9535) -> (-9.9504, -40.7072) construction
  line L2845 (-9.9504, -40.7072) -> (-10.1204, -40.7072) construction
  spline S864 degree 2 poles (-10.9496, -44.2355) (-10.9496, -44.4437) (-11.1578, -44.4437) knots 0 0 0 1 1 1
  line L2846 (-10.9496, -44.2355) -> (-10.9496, -44.4437) construction
  line L2847 (-10.9496, -44.4437) -> (-11.1578, -44.4437) construction
  spline S865 degree 2 poles (-11.1578, -44.4437) (-11.3659, -44.4437) (-11.3659, -44.2355) knots 0 0 0 1 1 1
  line L2848 (-11.1578, -44.4437) -> (-11.3659, -44.4437) construction
  line L2849 (-11.3659, -44.4437) -> (-11.3659, -44.2355) construction
  line L2850 (-11.3659, -44.2355) -> (-11.3659, -40.499)
  spline S866 degree 2 poles (-11.3659, -40.499) (-11.3659, -40.2909) (-11.1578, -40.2909) knots 0 0 0 1 1 1
  line L2851 (-11.3659, -40.499) -> (-11.3659, -40.2909) construction
  line L2852 (-11.3659, -40.2909) -> (-11.1578, -40.2909) construction
  line L2853 (-11.1578, -40.2909) -> (-10.1204, -40.2909)
  spline S867 degree 2 poles (-10.1204, -40.2909) (-9.777, -40.2909) (-9.2913, -40.7766) (-9.2913, -41.12) knots 0 0 0 1 2 2 2
  line L2854 (-10.1204, -40.2909) -> (-9.777, -40.2909) construction
  line L2855 (-9.777, -40.2909) -> (-9.2913, -40.7766) construction
  line L2856 (-9.2913, -40.7766) -> (-9.2913, -41.12) construction
  line L2857 (-9.2913, -41.12) -> (-9.2913, -42.369)
  spline S868 degree 2 poles (-9.2913, -42.369) (-9.2913, -42.7125) (-9.777, -43.1982) (-10.1204, -43.1982) knots 0 0 0 1 2 2 2
  line L2858 (-9.2913, -42.369) -> (-9.2913, -42.7125) construction
  line L2859 (-9.2913, -42.7125) -> (-9.777, -43.1982) construction
  line L2860 (-9.777, -43.1982) -> (-10.1204, -43.1982) construction
  spline S869 degree 2 poles (-7.2131, -42.7819) (-7.0431, -42.7819) (-6.8003, -42.5355) (-6.8003, -42.3655) knots 0 0 0 1 2 2 2
  line L2861 (-7.2131, -42.7819) -> (-7.0431, -42.7819) construction
  line L2862 (-7.0431, -42.7819) -> (-6.8003, -42.5355) construction
  line L2863 (-6.8003, -42.5355) -> (-6.8003, -42.3655) construction
  spline S870 degree 2 poles (-7.6295, -40.7072) (-7.7995, -40.7072) (-8.0423, -40.9535) (-8.0423, -41.1235) knots 0 0 0 1 2 2 2
  line L2864 (-7.6295, -40.7072) -> (-7.7995, -40.7072) construction
  line L2865 (-7.7995, -40.7072) -> (-8.0423, -40.9535) construction
  line L2866 (-8.0423, -40.9535) -> (-8.0423, -41.1235) construction
  line L2867 (-8.0423, -41.1235) -> (-8.0423, -42.3655)
  spline S871 degree 2 poles (-8.0423, -42.3655) (-8.0423, -42.5355) (-7.7995, -42.7819) (-7.6295, -42.7819) knots 0 0 0 1 2 2 2
  line L2868 (-8.0423, -42.3655) -> (-8.0423, -42.5355) construction
  line L2869 (-8.0423, -42.5355) -> (-7.7995, -42.7819) construction
  line L2870 (-7.7995, -42.7819) -> (-7.6295, -42.7819) construction
  line L2871 (-7.6295, -42.7819) -> (-7.2131, -42.7819)
  line L2872 (-7.2131, -43.1982) -> (-7.6295, -43.1982)
  spline S872 degree 2 poles (-7.6295, -43.1982) (-7.9694, -43.1982) (-8.4586, -42.7125) (-8.4586, -42.369) knots 0 0 0 1 2 2 2
  line L2873 (-7.6295, -43.1982) -> (-7.9694, -43.1982) construction
  line L2874 (-7.9694, -43.1982) -> (-8.4586, -42.7125) construction
  line L2875 (-8.4586, -42.7125) -> (-8.4586, -42.369) construction
  line L2876 (-8.4586, -42.369) -> (-8.4586, -41.12)
  spline S873 degree 2 poles (-8.4586, -41.12) (-8.4586, -40.7766) (-7.9694, -40.2909) (-7.6295, -40.2909) knots 0 0 0 1 2 2 2
  line L2877 (-8.4586, -41.12) -> (-8.4586, -40.7766) construction
  line L2878 (-8.4586, -40.7766) -> (-7.9694, -40.2909) construction
  line L2879 (-7.9694, -40.2909) -> (-7.6295, -40.2909) construction
  line L2880 (-7.6295, -40.2909) -> (-6.5921, -40.2909)
  spline S874 degree 2 poles (-6.5921, -40.2909) (-6.384, -40.2909) (-6.384, -40.499) knots 0 0 0 1 1 1
  line L2881 (-6.5921, -40.2909) -> (-6.384, -40.2909) construction
  line L2882 (-6.384, -40.2909) -> (-6.384, -40.499) construction
  line L2883 (-6.384, -40.499) -> (-6.384, -42.3621)
  spline S875 degree 2 poles (-6.384, -42.3621) (-6.384, -42.6743) (-6.0925, -42.7992) knots 0 0 0 1 1 1
  line L2884 (-6.384, -42.3621) -> (-6.384, -42.6743) construction
  line L2885 (-6.384, -42.6743) -> (-6.0925, -42.7992) construction
  spline S876 degree 2 poles (-6.0925, -42.7992) (-5.9642, -42.8512) (-5.9642, -42.9831) knots 0 0 0 1 1 1
  line L2886 (-6.0925, -42.7992) -> (-5.9642, -42.8512) construction
  line L2887 (-5.9642, -42.8512) -> (-5.9642, -42.9831) construction
  spline S877 degree 2 poles (-5.9642, -42.9831) (-5.9642, -43.0698) (-6.0821, -43.2016) (-6.1689, -43.2016) knots 0 0 0 1 2 2 2
  line L2888 (-5.9642, -42.9831) -> (-5.9642, -43.0698) construction
  line L2889 (-5.9642, -43.0698) -> (-6.0821, -43.2016) construction
  line L2890 (-6.0821, -43.2016) -> (-6.1689, -43.2016) construction
  spline S878 degree 2 poles (-6.1689, -43.2016) (-6.214, -43.2016) (-6.2591, -43.1808) knots 0 0 0 1 1 1
  line L2891 (-6.1689, -43.2016) -> (-6.214, -43.2016) construction
  line L2892 (-6.214, -43.2016) -> (-6.2591, -43.1808) construction
  spline S879 degree 2 poles (-6.2591, -43.1808) (-6.4672, -43.0906) (-6.5956, -42.9241) knots 0 0 0 1 1 1
  line L2893 (-6.2591, -43.1808) -> (-6.4672, -43.0906) construction
  line L2894 (-6.4672, -43.0906) -> (-6.5956, -42.9241) construction
  spline S880 degree 2 poles (-6.5956, -42.9241) (-6.8454, -43.1982) (-7.2131, -43.1982) knots 0 0 0 1 1 1
  line L2895 (-6.5956, -42.9241) -> (-6.8454, -43.1982) construction
  line L2896 (-6.8454, -43.1982) -> (-7.2131, -43.1982) construction
  line L2897 (-5.135, -39.7913) -> (-5.135, -40.4366)
  spline S881 degree 2 poles (-5.135, -40.4366) (-4.9719, -40.3325) (-4.7222, -40.1486) knots 0 0 0 1 1 1
  line L2898 (-5.135, -40.4366) -> (-4.9719, -40.3325) construction
  line L2899 (-4.9719, -40.3325) -> (-4.7222, -40.1486) construction
  spline S882 degree 2 poles (-4.7222, -40.1486) (-4.4724, -39.9474) (-4.4724, -39.7913) knots 0 0 0 1 1 1
  line L2900 (-4.7222, -40.1486) -> (-4.4724, -39.9474) construction
  line L2901 (-4.4724, -39.9474) -> (-4.4724, -39.7913) construction
  spline S883 degree 2 poles (-4.4724, -39.7913) (-4.4724, -39.6317) (-4.5764, -39.5415) knots 0 0 0 1 1 1
  line L2902 (-4.4724, -39.7913) -> (-4.4724, -39.6317) construction
  line L2903 (-4.4724, -39.6317) -> (-4.5764, -39.5415) construction
  spline S884 degree 2 poles (-4.5764, -39.5415) (-4.6701, -39.4617) (-4.8019, -39.4617) knots 0 0 0 1 1 1
  line L2904 (-4.5764, -39.5415) -> (-4.6701, -39.4617) construction
  line L2905 (-4.6701, -39.4617) -> (-4.8019, -39.4617) construction
  spline S885 degree 2 poles (-4.8019, -39.4617) (-4.9407, -39.4617) (-5.0309, -39.5415) knots 0 0 0 1 1 1
  line L2906 (-4.8019, -39.4617) -> (-4.9407, -39.4617) construction
  line L2907 (-4.9407, -39.4617) -> (-5.0309, -39.5415) construction
  spline S886 degree 2 poles (-5.0309, -39.5415) (-5.135, -39.6317) (-5.135, -39.7913) knots 0 0 0 1 1 1
  line L2908 (-5.0309, -39.5415) -> (-5.135, -39.6317) construction
  line L2909 (-5.135, -39.6317) -> (-5.135, -39.7913) construction
  spline S887 degree 2 poles (-4.3058, -42.7819) (-4.1358, -42.7819) (-3.893, -42.5355) (-3.893, -42.3655) knots 0 0 0 1 2 2 2
  line L2910 (-4.3058, -42.7819) -> (-4.1358, -42.7819) construction
  line L2911 (-4.1358, -42.7819) -> (-3.893, -42.5355) construction
  line L2912 (-3.893, -42.5355) -> (-3.893, -42.3655) construction
  line L2913 (-3.893, -42.3655) -> (-3.893, -41.12)
  spline S888 degree 2 poles (-3.893, -41.12) (-3.893, -40.95) (-4.1358, -40.7037) (-4.3058, -40.7037) knots 0 0 0 1 2 2 2
  line L2914 (-3.893, -41.12) -> (-3.893, -40.95) construction
  line L2915 (-3.893, -40.95) -> (-4.1358, -40.7037) construction
  line L2916 (-4.1358, -40.7037) -> (-4.3058, -40.7037) construction
  line L2917 (-4.3058, -40.7037) -> (-4.7222, -40.7037)
  spline S889 degree 2 poles (-4.7222, -40.7037) (-4.8922, -40.7037) (-5.135, -40.95) (-5.135, -41.12) knots 0 0 0 1 2 2 2
  line L2918 (-4.7222, -40.7037) -> (-4.8922, -40.7037) construction
  line L2919 (-4.8922, -40.7037) -> (-5.135, -40.95) construction
  line L2920 (-5.135, -40.95) -> (-5.135, -41.12) construction
  line L2921 (-5.135, -41.12) -> (-5.135, -42.3655)
  spline S890 degree 2 poles (-5.135, -42.3655) (-5.135, -42.5355) (-4.8922, -42.7819) (-4.7222, -42.7819) knots 0 0 0 1 2 2 2
  line L2922 (-5.135, -42.3655) -> (-5.135, -42.5355) construction
  line L2923 (-5.135, -42.5355) -> (-4.8922, -42.7819) construction
  line L2924 (-4.8922, -42.7819) -> (-4.7222, -42.7819) construction
  line L2925 (-4.7222, -42.7819) -> (-4.3058, -42.7819)
  spline S891 degree 2 poles (-3.6814, -40.5407) (-3.4767, -40.7592) (-3.4767, -41.12) knots 0 0 0 1 1 1
  line L2926 (-3.6814, -40.5407) -> (-3.4767, -40.7592) construction
  line L2927 (-3.4767, -40.7592) -> (-3.4767, -41.12) construction
  line L2928 (-3.4767, -41.12) -> (-3.4767, -42.369)
  spline S892 degree 2 poles (-3.4767, -42.369) (-3.4767, -42.7125) (-3.9624, -43.1982) (-4.3058, -43.1982) knots 0 0 0 1 2 2 2
  line L2929 (-3.4767, -42.369) -> (-3.4767, -42.7125) construction
  line L2930 (-3.4767, -42.7125) -> (-3.9624, -43.1982) construction
  line L2931 (-3.9624, -43.1982) -> (-4.3058, -43.1982) construction
  line L2932 (-4.3058, -43.1982) -> (-4.7222, -43.1982)
  spline S893 degree 2 poles (-4.7222, -43.1982) (-5.0621, -43.1982) (-5.5513, -42.7125) (-5.5513, -42.369) knots 0 0 0 1 2 2 2
  line L2933 (-4.7222, -43.1982) -> (-5.0621, -43.1982) construction
  line L2934 (-5.0621, -43.1982) -> (-5.5513, -42.7125) construction
  line L2935 (-5.5513, -42.7125) -> (-5.5513, -42.369) construction
  line L2936 (-5.5513, -42.369) -> (-5.5513, -39.7913)
  spline S894 degree 2 poles (-5.5513, -39.7913) (-5.5513, -39.4409) (-5.3189, -39.2327) knots 0 0 0 1 1 1
  line L2937 (-5.5513, -39.7913) -> (-5.5513, -39.4409) construction
  line L2938 (-5.5513, -39.4409) -> (-5.3189, -39.2327) construction
  spline S895 degree 2 poles (-5.3189, -39.2327) (-5.1073, -39.0454) (-4.7985, -39.0454) knots 0 0 0 1 1 1
  line L2939 (-5.3189, -39.2327) -> (-5.1073, -39.0454) construction
  line L2940 (-5.1073, -39.0454) -> (-4.7985, -39.0454) construction
  spline S896 degree 2 poles (-4.7985, -39.0454) (-4.4966, -39.0454) (-4.2885, -39.2293) knots 0 0 0 1 1 1
  line L2941 (-4.7985, -39.0454) -> (-4.4966, -39.0454) construction
  line L2942 (-4.4966, -39.0454) -> (-4.2885, -39.2293) construction
  spline S897 degree 2 poles (-4.2885, -39.2293) (-4.056, -39.4374) (-4.056, -39.7878) knots 0 0 0 1 1 1
  line L2943 (-4.2885, -39.2293) -> (-4.056, -39.4374) construction
  line L2944 (-4.056, -39.4374) -> (-4.056, -39.7878) construction
  spline S898 degree 2 poles (-4.056, -39.7878) (-4.056, -40.1382) (-4.3058, -40.3048) knots 0 0 0 1 1 1
  line L2945 (-4.056, -39.7878) -> (-4.056, -40.1382) construction
  line L2946 (-4.056, -40.1382) -> (-4.3058, -40.3048) construction
  spline S899 degree 2 poles (-4.3058, -40.3048) (-3.9034, -40.3048) (-3.6814, -40.5407) knots 0 0 0 1 1 1
  line L2947 (-4.3058, -40.3048) -> (-3.9034, -40.3048) construction
  line L2948 (-3.9034, -40.3048) -> (-3.6814, -40.5407) construction
  spline S900 degree 2 poles (1.0924, -40.7072) (0.8982, -40.7072) (0.6796, -40.95) (0.6796, -41.12) knots 0 0 0 1 2 2 2
  line L2949 (1.0924, -40.7072) -> (0.8982, -40.7072) construction
  line L2950 (0.8982, -40.7072) -> (0.6796, -40.95) construction
  line L2951 (0.6796, -40.95) -> (0.6796, -41.12) construction
  spline S901 degree 2 poles (0.6796, -41.12) (0.6796, -41.29) (0.7837, -41.408) knots 0 0 0 1 1 1
  line L2952 (0.6796, -41.12) -> (0.6796, -41.29) construction
  line L2953 (0.6796, -41.29) -> (0.7837, -41.408) construction
  spline S902 degree 2 poles (0.7837, -41.408) (0.8982, -41.5364) (1.0924, -41.5364) knots 0 0 0 1 1 1
  line L2954 (0.7837, -41.408) -> (0.8982, -41.5364) construction
  line L2955 (0.8982, -41.5364) -> (1.0924, -41.5364) construction
  spline S903 degree 2 poles (0.6449, -43.1045) (0.5825, -43.2016) (0.4784, -43.2016) knots 0 0 0 1 1 1
  line L2956 (0.6449, -43.1045) -> (0.5825, -43.2016) construction
  line L2957 (0.5825, -43.2016) -> (0.4784, -43.2016) construction
  spline S904 degree 2 poles (0.4784, -43.2016) (0.3916, -43.2016) (0.2598, -43.0767) (0.2598, -42.9935) knots 0 0 0 1 2 2 2
  line L2958 (0.4784, -43.2016) -> (0.3916, -43.2016) construction
  line L2959 (0.3916, -43.2016) -> (0.2598, -43.0767) construction
  line L2960 (0.2598, -43.0767) -> (0.2598, -42.9935) construction
  spline S905 degree 2 poles (0.2598, -42.9935) (0.2598, -42.931) (0.298, -42.8755) knots 0 0 0 1 1 1
  line L2961 (0.2598, -42.9935) -> (0.2598, -42.931) construction
  line L2962 (0.2598, -42.931) -> (0.298, -42.8755) construction
  line L2963 (0.298, -42.8755) -> (0.9224, -41.9388)
  spline S906 degree 2 poles (0.9224, -41.9388) (0.6102, -41.8868) (0.4263, -41.6404) knots 0 0 0 1 1 1
  line L2964 (0.9224, -41.9388) -> (0.6102, -41.8868) construction
  line L2965 (0.6102, -41.8868) -> (0.4263, -41.6404) construction
  spline S907 degree 2 poles (0.4263, -41.6404) (0.2633, -41.4184) (0.2633, -41.12) knots 0 0 0 1 1 1
  line L2966 (0.4263, -41.6404) -> (0.2633, -41.4184) construction
  line L2967 (0.2633, -41.4184) -> (0.2633, -41.12) construction
  spline S908 degree 2 poles (0.2633, -41.12) (0.2633, -40.7835) (0.4714, -40.5511) knots 0 0 0 1 1 1
  line L2968 (0.2633, -41.12) -> (0.2633, -40.7835) construction
  line L2969 (0.2633, -40.7835) -> (0.4714, -40.5511) construction
  spline S909 degree 2 poles (0.4714, -40.5511) (0.7004, -40.2909) (1.0924, -40.2909) knots 0 0 0 1 1 1
  line L2970 (0.4714, -40.5511) -> (0.7004, -40.2909) construction
  line L2971 (0.7004, -40.2909) -> (1.0924, -40.2909) construction
  line L2972 (1.0924, -40.2909) -> (2.1298, -40.2909)
  spline S910 degree 2 poles (2.1298, -40.2909) (2.3379, -40.2909) (2.3379, -40.499) knots 0 0 0 1 1 1
  line L2973 (2.1298, -40.2909) -> (2.3379, -40.2909) construction
  line L2974 (2.3379, -40.2909) -> (2.3379, -40.499) construction
  line L2975 (2.3379, -40.499) -> (2.3379, -42.99)
  spline S911 degree 2 poles (2.3379, -42.99) (2.3379, -43.1982) (2.1298, -43.1982) knots 0 0 0 1 1 1
  line L2976 (2.3379, -42.99) -> (2.3379, -43.1982) construction
  line L2977 (2.3379, -43.1982) -> (2.1298, -43.1982) construction
  spline S912 degree 2 poles (2.1298, -43.1982) (1.9216, -43.1982) (1.9216, -42.99) knots 0 0 0 1 1 1
  line L2978 (2.1298, -43.1982) -> (1.9216, -43.1982) construction
  line L2979 (1.9216, -43.1982) -> (1.9216, -42.99) construction